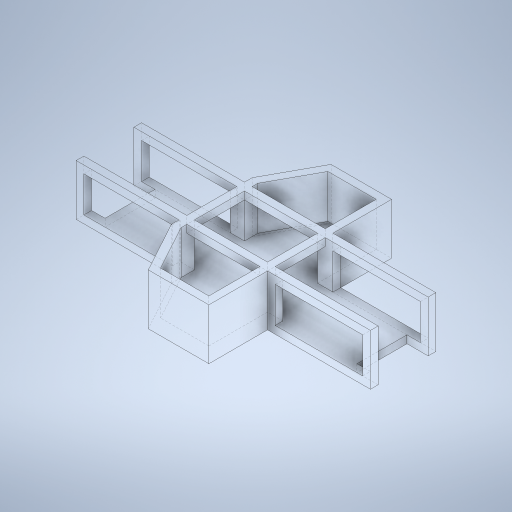
# Autodesk Inventor part: body
Saved by Autodesk Inventor 2023 (Build 270158000, 158)
## iProperties
Created: 2024-02-05
Part Number: body
Material: 일반
Document SubType Name: Modeling
Designer: ps737
Density: 1 g/cm^3
Appearance: 기본값
Author: ps737
Autodesk Inventor part; units mm, degrees
ref_plane "YZ Plane" through (0, 0, 0) normal (1, 0, 0) x (0, 1, 0)
ref_plane "XZ Plane" through (0, 0, 0) normal (0, 1, 0) x (-1, 0, 0)
ref_plane "XY Plane" through (0, 0, 0) normal (0, 0, 1) x (1, 0, 0)
sketch "스케치1" plane through (0, 0, 0) normal (0, 1, 0) x (-1, 0, 0)
  line L0 (0, 475) -> (0, -475)
  line L1 (0, 475) -> (315, 475)
  line L2 (460, 170) -> (460, -170)
  line L3 (315, -475) -> (0, -475)
  line L4 (0, 0) -> (678.9617, 0) construction
  line L5 (460, 170) -> (995, 170)
  line L6 (995, -170) -> (460, -170)
  line L7 (460, 130) -> (995, 130)
  line L8 (995, -130) -> (460, -130)
  line L9 (995, 170) -> (995, 130)
  line L10 (995, -130) -> (995, -170)
  line L11 (0, 170) -> (-535, 170)
  line L12 (-535, -170) -> (0, -170)
  line L13 (-10, 130) -> (-535, 130)
  line L14 (-535, -130) -> (-10, -130)
  line L15 (-535, 170) -> (-535, 130)
  line L16 (-535, -130) -> (-535, -170)
  line L17 (460, 170) -> (460, 210)
  line L18 (460, -170) -> (460, -210)
  line L19 (460, 210) -> (315, 475)
  line L20 (460, -210) -> (315, -475)
  line L21 (420, 170) -> (420, 199.7721)
  line L22 (420, 199.7721) -> (291.2904, 435)
  line L23 (291.2904, 435) -> (40, 435)
  line L24 (40, 435) -> (40, -435)
  line L25 (40, -435) -> (291.2904, -435)
  line L26 (291.2904, -435) -> (420, -199.7721)
  line L27 (420, -199.7721) -> (420, 170)
  line L28 (460, -170) -> (0, -170)
  line L29 (-10, -130) -> (460, -130)
  line L30 (460, 130) -> (-10, 130)
  line L31 (460, 170) -> (0, 170)
  point P0 (460, 0)
  point P1 (995, -150)
  point P2 (-535, -150)
  point P3 (0, 130)
  point P4 (0, -130)
  point P5 (460, -190)
  point P6 (0, -130)
  point P7 (0, 130)
  dimension "d1" = 315
  dimension "d2" = 950
  dimension "d3" = 340
  dimension "d4" = 535
  dimension "d5" = 40
  dimension "d6" = 40
  dimension "d7" = 535
  dimension "d8" = 40
  dimension "d9" = 40
  dimension "d10" = 340
  dimension "d11" = 130
  dimension "d12" = 460
  dimension "d13" = 535
  dimension "d14" = 40
  dimension "d15" = 40
  dimension "d16" = 315
  dimension "d17" = 535
  dimension "d32" = 40
  dimension "d42" = 40
  constraints: 64 end point, 9 perpendicular, 5 midpoint, 5 point on line, 4 horizontal, 3 vertical, 2 parallel, 1 coincident, 5 other
  measures "d1" distance from line of L1.end L0
  measures "d2" distance between parallel lines of L3 L1
  measures "d3" distance of L2.end L2.start
  measures "d4" distance of L2.start L5.end
  measures "d5" distance between parallel lines of L5 L7
  measures "d6" distance between parallel lines of L6 L8
  measures "d7" distance of L11.start L11.end
  measures "d8" distance between parallel lines of L11 L13
  measures "d9" distance between parallel lines of L12 L14
  measures "d10" distance between parallel lines of L12 L11
  measures "d11" distance between parallel lines of L4 L13
  measures "d12" distance between parallel lines of L0 L2
  measures "d13" distance from line of L2 point (995, -150)
  measures "d14" distance of L2.start L17.end
  measures "d15" distance of L2.end L18.end
  measures "d16" distance from line of L0 L3.start
  measures "d17" distance from line of L0 point (-535, -150)
  measures "d32" distance between parallel lines of L20 L26
  measures "d42" distance from line of point (460, -190) L27
extrude "돌출1" add sketch "스케치1" along normal mid plane 265
sketch "스케치2" plane through (-995, 132.5, 170) normal (0, 0, 1) x (1, 0, 0)
  line L0 (535, -265) -> (535, 0) projected
  line L1 (0, 0) -> (535, 0) projected
  line L2 (0, -265) -> (0, 0) projected
  line L3 (535, -265) -> (0, -265) projected
  line L4 (1530, -265) -> (1530, 0) projected
  line L5 (995, 0) -> (1530, 0) projected
  line L6 (995, -265) -> (995, 0) projected
  line L7 (1530, -265) -> (995, -265) projected
  line L8 (500, -40) -> (500, -225)
  line L9 (535, -225) -> (0, -225)
  line L10 (40, -225) -> (40, -40)
  line L11 (40, -40) -> (535, -40)
  line L12 (1490, -40) -> (1490, -225)
  line L13 (1530, -225) -> (995, -225)
  line L14 (1035, -225) -> (1035, -40)
  line L15 (995, -40) -> (1490, -40)
  point P0 (995, -132.5)
  dimension "d20" = 40
  dimension "d21" = 40
  dimension "d30" = 185
  dimension "d31" = 40
  constraints: 16 end point, 12 point on line
  measures "d20" distance between parallel lines of L1 L11
  measures "d21" distance between parallel lines of L5 L15
  measures "d30" distance between parallel lines of L9 L11
  measures "d31" distance between parallel lines of L2 L10
extrude "돌출2" cut sketch "스케치2" against normal blind 8000 contours L9 L10 L11 L8 | L13 L14 L15 L12
extrude "돌출3" add sketch "스케치2" against normal blind 340 contours L3 L2 L9 L0 | L7 L6 L13 L4
sketch "스케치3" plane through (-955, -92.5, 170) normal (0, 1, 0) x (1, 0, 0)
  line L0 (70, 300) -> (70, 40)
  line L1 (1490, 300) -> (1380, 300)
  line L2 (1380, 300) -> (1380, 40)
  line L3 (1490, 0) -> (1490, 40) projected
  line L4 (1380, 40) -> (1490, 40)
  line L5 (70, 40) -> (-40, 40)
  line L6 (-40, 0) -> (-40, 340) projected
  line L7 (1490, 40) -> (1490, 300) projected
  line L8 (-40, 300) -> (0, 300) projected
  line L9 (-40, 300) -> (70, 300)
  point P0 (955, 170)
  dimension "d26" = 110
  dimension "d43" = 110
  constraints: 12 end point, 2 horizontal, 1 collinear, 1 perpendicular, 1 point on line
  measures "d26" distance of L8.start L0.start
  measures "d43" distance between parallel lines of L7 L2
sketch "스케치4" plane through (0, 132.5, 0) normal (0, 1, 0) x (1, 0, 0)
  line L0 (0, -475) -> (0, -170) projected
  line L1 (0, -170) -> (535, -170) projected
  line L2 (535, -170) -> (535, -130) projected
  line L3 (535, -130) -> (0, -130) projected
  line L4 (0, 170) -> (0, 475) projected
  line L5 (0, 475) -> (-315, 475) projected
  line L6 (-315, 475) -> (-460, 210) projected
  line L7 (-460, 210) -> (-460, 170) projected
  line L8 (-460, 170) -> (-995, 170) projected
  line L9 (-995, 170) -> (-995, 130) projected
  line L10 (-995, 130) -> (-460, 130) projected
  line L11 (-460, 130) -> (-460, -130) projected
  line L12 (-460, -130) -> (-995, -130) projected
  line L13 (-995, -130) -> (-995, -170) projected
  line L14 (-995, -170) -> (-460, -170) projected
  line L15 (-460, -170) -> (-460, -210) projected
  line L16 (-460, -210) -> (-315, -475) projected
  line L17 (-315, -475) -> (0, -475) projected
  line L18 (-291.2904, -435) -> (-420, -199.7721)
  line L19 (-420, -199.7721) -> (-420, -170)
  line L20 (-420, -170) -> (-420, 130)
  line L21 (-420, 130) -> (-420, 199.7721)
  line L22 (-420, 199.7721) -> (-291.2904, 435)
  line L23 (-291.2904, 435) -> (-40, 435)
  line L24 (-40, 435) -> (-40, 170)
  line L25 (-40, 170) -> (-40, -130)
  line L26 (-40, -130) -> (-40, -435)
  line L27 (-40, -435) -> (-291.2904, -435)
  line L28 (-460, -170) -> (0, -170)
  line L29 (-460, -130) -> (0, -130)
  line L30 (-460, 170) -> (0, 170)
  line L31 (0, -130) -> (0, 130) projected
  line L32 (0, 130) -> (535, 130) projected
  line L33 (535, 130) -> (535, 170) projected
  line L34 (535, 170) -> (0, 170) projected
  line L35 (0, 130) -> (-460, 130)
  point P0 (0, 0)
  point P1 (-420, 170)
  point P2 (-420, -130)
  point P3 (-40, -170)
  point P4 (-420, -170)
  point P5 (-165.6452, 435)
  point P6 (-40, 130)
  point P7 (-420, 130)
  dimension "d33" = 40
  dimension "d46" = 40
  dimension "d47" = 90
  dimension "d48" = 265
  constraints: 28 end point, 2 horizontal, 1 midpoint, 1 parallel, 1 point on line, 7 other
  measures "d33" distance between parallel lines of L16 L18
  measures "d46" distance between parallel lines of L17 L27
  measures "d47" angle of L23 L24
  measures "d48" distance from line of point (-165.645, 435) L30
sketch "스케치5" plane through (-460, 132.5, -130) normal (-1, 0, 0) x (0, 0, 1)
  line L0 (0, 0) -> (260, 0) projected
  line L1 (0, -225) -> (260, -225) projected
  line L2 (0, -40) -> (260, -40)
  line L3 (0, -225) -> (0, 0) projected
  line L4 (260, -225) -> (260, 0) projected
  point P0 (130, -132.5)
  point P1 (0, -265)
  point P2 (260, -265)
  dimension "d36" = 40
  constraints: 2 end point, 1 parallel
  measures "d36" distance between parallel lines of L0 L2
extrude "돌출6" cut sketch "스케치5" against normal blind 1000 contours L2 L4 L1 L3
ref_plane "작업 평면1" through (-420, 132.5, 170) normal (0, 0, 1) x (1, 0, 0)
sketch "스케치7" plane through (-420, 132.5, 170) normal (0, 0, 1) x (1, 0, 0)
  line L0 (0, 0) -> (380, 0) projected
  line L1 (0, -40) -> (390, -40)
  line L2 (0, 0) -> (380, 0) projected
  line L3 (0, 0) -> (0, -225) projected
  line L4 (0, -225) -> (380, -225) projected
  line L5 (380, 0) -> (380, -225) projected
  point P0 (420, -132.5)
  point P1 (380, -40)
  dimension "d39" = 40
  constraints: 2 end point, 1 parallel
  measures "d39" distance between parallel lines of L0 L1
extrude "돌출7" cut sketch "스케치7" against normal blind 350 contours L1 L5 L4 L3
extrude "돌출8" cut sketch "스케치3" against normal blind 265
extrude "돌출9" cut sketch "스케치4" against normal blind 225 contours L26 L27 L18 L19 L28 | L29 L20 L35 L25 | L30 L21 L22 L23 L24
